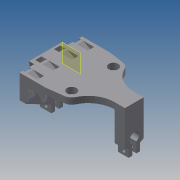
# Autodesk Inventor part: rollerBetter
Saved by Autodesk Inventor 2014 (Build 180170000, 170)
## iProperties
Created: 2014-01-09
Part Number: rollerBetter
Material: Generic
Document SubType Name: Modeling
Designer: Peele
Density: 1 g/cm^3
Appearance: Default
Author: Peele
Autodesk Inventor part; units mm, degrees
ref_plane "YZ Plane" through (0, 0, 0) normal (1, 0, 0) x (0, 1, 0)
ref_plane "XZ Plane" through (0, 0, 0) normal (0, 1, 0) x (-1, 0, 0)
ref_plane "XY Plane" through (0, 0, 0) normal (0, 0, 1) x (1, 0, 0)
sketch "Sketch1" plane through (0, 0, 0) normal (0, 1, 0) x (-1, 0, 0)
  circle A0 centre (0, 20) radius 14.875 construction
  circle A1 centre (0, 20) radius 13.26 construction
  circle A2 centre (0, -20) radius 14.875 construction
  circle A3 centre (0, -20) radius 13.26 construction
  circle A4 centre (0, -20) radius 4.5
  circle A5 centre (0, 20) radius 4.5
  line L0 (0, -20) -> (0, 0) construction
  line L1 (0, 0) -> (0, 20) construction
  arc A6 (-1.036149, 27.932616) -> (-7.232355, 23.419508) centre (0, 20) ccw
  arc A7 (-7.232355, -23.419508) -> (-1.155827, -27.916064) centre (0, -20) ccw
  line L2 (25, 30) -> (40, 30)
  line L3 (40, 30) -> (40, -30)
  line L4 (40, -30) -> (25, -30)
  line L5 (25, -30) -> (25, 30) construction
  line L6 (0, 0) -> (40, 0) construction
  arc A8 (-7.232355, -23.419508) -> (-30, -9) centre (-30, -34.184211) ccw
  arc A9 (-30, 9) -> (-7.232355, 23.419508) centre (-30, 34.184211) ccw
  line L7 (-30, 9) -> (-40, 9)
  line L8 (-40, 9) -> (-40, -9)
  line L9 (-40, -9) -> (-30, -9)
  line L10 (0, 0) -> (-40, 0) construction
  line L11 (25, 30) -> (15, 30)
  arc A10 (15, 30) -> (14.584682, 29.972991) centre (15, 26.793371) ccw
  line L12 (14.584682, 29.972991) -> (-1.036149, 27.932616)
  line L13 (-1.155827, -27.916064) -> (11.253156, -29.727904)
  line L14 (25, -30) -> (15, -30)
  arc A11 (11.253156, -29.727904) -> (15, -30) centre (15, -4.066406) ccw
  dimension "d0" = 29.75
  dimension "d1" = 26.52
  dimension "d2" = 40
  dimension "d3" = 9
  dimension "d4" = 16
  dimension "d5" = 60
  dimension "d6" = 15
  dimension "d7" = 25
  dimension "d66" = 10
  dimension "d67" = 18
  dimension "d68" = 40
  dimension "d87" = 10
  constraints: 30 end point, 13 point on circle, 11 centre point, 11 tangent, 6 coincident, 6 parallel, 3 equal length, 3 equal radius, 3 horizontal, 2 midpoint, 2 perpendicular, 1 collinear, 1 vertical, 4 other
  measures "d0" diameter of A0
  measures "d1" diameter of A1
  measures "d2" distance of point (0, -20) A0.centre
  measures "d3" diameter of A5
  measures "d4" diameter of A6
  measures "d5" distance of L2.end L3.end
  measures "d6" distance of L2.start L2.end
  measures "d7" distance from line of A0.centre L5
  measures "d66" distance of L7.start L7.end
  measures "d67" distance of L7.end L8.end
  measures "d68" distance between parallel lines of L8 L0
  measures "d87" distance of L2.start L11.end
extrude "Extrusion1" add sketch "Sketch1" along normal blind 6
sketch "Sketch2" plane through (0, 0, 0) normal (0, 0, 1) x (1, 0, 0)
  line L0 (-40, 0) -> (-34, 0)
  line L1 (-34, -8.5) -> (-34, -40)
  line L2 (-34, -40) -> (-40, -40)
  line L3 (-40, -40) -> (-40, 0)
  circle A0 centre (-26, -8.5) radius 8
  line L4 (-34, 0) -> (-15.298824, 0)
  line L5 (-15.298824, 0) -> (-18.298824, -10.666076)
  line L6 (7.232355, 0) -> (1.036149, 0)
  point P0 (0, 0)
  point P1 (4.134252, 0)
  dimension "d11" = 6
  dimension "d12" = 40
  dimension "d13" = 16
  dimension "d15" = 8.5
  dimension "d16" = 3
  constraints: 12 end point, 2 parallel, 2 perpendicular, 2 point on circle, 2 tangent, 1 centre point, 1 coincident, 1 horizontal, 1 midpoint
  measures "d11" distance of L1.end L2.end
  measures "d12" distance of L2.end L0.start
  measures "d13" diameter of A0
  measures "d15" distance from line of A0.centre L4
  measures "d16" horizontal distance of L4.end L5.end
extrude "Extrusion11" add sketch "Sketch2" along normal mid plane 60 contours L0 L4 L5 A0 L1 L2 L3
sketch "Sketch11" plane through (0, 0, 0) normal (0, 0, 1) x (1, 0, 0)
  line L0 (40, 0) -> (30, 0)
  line L1 (30, 0) -> (30, -40)
  line L2 (30, -40) -> (40, -40)
  line L3 (40, -40) -> (40, 0)
  line L4 (40, 0) -> (40, 6) projected
  line L5 (-34, -40) -> (-40, -40) projected
  point P0 (0, 0)
  dimension "d71" = 10
  constraints: 8 end point, 2 collinear, 2 parallel, 1 horizontal, 1 perpendicular
  measures "d71" distance of L1.end L2.end
extrude "Extrusion12" add sketch "Sketch11" along normal mid plane 18
sketch "Sketch3" plane through (-25, 6, -30) normal (0, 0, -1) x (-1, 0, 0)
  arc A0 (9, -14.5) -> (-6.701176, -16.666076) centre (1, -14.5) ccw
  arc A1 (7.402553, -13.378697) -> (-5.128468, -16.666076) centre (1, -14.5) ccw
  arc A2 (9, -14.5) -> (-6.701176, -16.666076) centre (1, -14.5) ccw
  line L0 (7.402553, -13.378697) -> (9, -22.5)
  line L1 (9, -22.5) -> (9, -14.5)
  line L2 (-6.701176, -16.666076) -> (-5.128468, -16.666076)
  point P0 (-25, -6)
  point P1 (-5.914822, -16.666076)
  dimension "d74" = 1.5
  dimension "d75" = 8
  constraints: 6 end point, 4 point on circle, 3 tangent, 2 centre point, 2 concentric, 1 coincident, 1 midpoint, 1 perpendicular, 1 point on line, 1 vertical
  measures "d74" radial gap between concentric circles of A0 A1
  measures "d75" distance of L0.end L1.end
extrude "Extrusion13" add sketch "Sketch3" against normal blind 3
mirror "Mirror1" about plane through (0, 0, 0) normal (0, 0, 1) of "Extrusion13"
sketch "Sketch13" plane through (0, 0, 0) normal (0, 0, 1) x (1, 0, 0)
  line L0 (-34, -16.5) -> (-32.402553, -7.378697)
  line L1 (-19.871532, -10.666076) -> (-18.298824, -10.666076)
  line L2 (-18.298824, -10.666076) -> (-15.298824, 0)
  line L3 (-15.298824, 0) -> (-34, 0)
  line L4 (-34, 0) -> (-34, -16.5)
  arc A0 (-19.871532, -10.666076) -> (-32.402553, -7.378697) centre (-26, -8.5) ccw
  arc A1 (-19.871532, -10.666076) -> (-32.402553, -7.378697) centre (-26, -8.5) ccw
  line L5 (-19.871532, -10.666076) -> (-18.298824, -10.666076)
  line L6 (-15.298824, 0) -> (-18.298824, -10.666076)
  line L7 (-15, 0) -> (-15.298824, 0)
  line L8 (-34, -16.5) -> (-34, -40)
  line L9 (-34, -16.5) -> (-32.402553, -7.378697)
  point P0 (0, 0)
  point P1 (-25, 0)
  point P2 (-40, 0)
  constraints: 10 end point, 5 collinear, 2 concentric, 2 point on circle, 1 centre point, 1 horizontal, 1 parallel
extrude "Extrusion14" add sketch "Sketch13" along normal mid plane 4
sketch "Sketch4" plane through (-40, 6, 30) normal (0, 0, 1) x (1, 0, 0)
  arc A0 (20.468886, -13.854567) -> (22.467566, -13.806595) centre (21.467571, -13.80331) ccw
  line L0 (24.701176, -6) -> (21.701176, -16.666076)
  arc A1 (20.128468, -16.666076) -> (7.597447, -13.378697) centre (14, -14.5) ccw
  line L1 (20.468886, -13.854567) -> (16.501696, -13.854567)
  line L2 (16.501696, -13.854567) -> (16.051575, -20.057074)
  line L3 (16.051575, -20.057074) -> (25.203638, -20.057074)
  line L4 (25.203638, -20.057074) -> (25.203638, -13.806595)
  line L5 (25.203638, -13.806595) -> (22.467566, -13.806595)
  point P0 (40, -6)
  dimension "d78" = 1
  constraints: 10 end point, 2 parallel, 2 point on circle, 2 tangent, 1 centre point, 1 horizontal, 1 perpendicular
  measures "d78" radius of A0
sketch "Sketch4 outline for Extrusion4" plane through (-40, 6, 30) normal (0, 0, 1) x (1, 0, 0)
  arc A0 (20.468886, -13.854567) -> (22.467566, -13.806595) centre (21.467571, -13.80331) ccw
  line L0 (22.467566, -13.806595) -> (25.203638, -13.806595)
  line L1 (25.203638, -13.806595) -> (25.203638, -20.057074)
  line L2 (25.203638, -20.057074) -> (16.051575, -20.057074)
  line L3 (16.051575, -20.057074) -> (16.501696, -13.854567)
  line L4 (16.501696, -13.854567) -> (20.468886, -13.854567)
extrude "Extrusion4" cut sketch "Sketch4 outline for Extrusion4" against normal blind 63.8125
sketch "Sketch5" plane through (-40, 6, -30) normal (-1, 0, 0) x (0, 0, 1)
  circle A0 centre (30, -29) radius 4.5
  arc A1 (31.363961, -41.636039) -> (31.363961, -41.636039) centre (41.970563, -52.242641) ccw
  arc A2 (18.636039, -41.636039) -> (18.636039, -41.636039) centre (8.029437, -52.242641) ccw
  line L0 (60, -46) -> (60, 0)
  line L1 (0, 0) -> (60, 0)
  line L2 (0, -46) -> (0, 0)
  line L3 (60, -23) -> (0, -23) construction
  line L4 (30, 0) -> (30, -29) construction
  arc A3 (26.082937, -36.543648) -> (33.917063, -36.543648) centre (30, -29) ccw
  line L5 (0, -23) -> (26.082937, -36.543648)
  line L6 (33.917063, -36.543648) -> (60, -23)
  line L7 (0, -46) -> (60, -46)
  line L8 (0, -23) -> (0, -46)
  line L9 (60, -46) -> (60, -23)
  line L10 (60, -46) -> (0, -46)
  dimension "d28" = 9
  dimension "d81" = 23
  dimension "d82" = 6
  dimension "d83" = 4
  constraints: 14 end point, 6 point on circle, 4 centre point, 4 midpoint, 3 collinear, 2 coincident, 2 tangent, 1 equal length, 1 equal radius, 1 horizontal, 1 vertical
  measures "d28" diameter of A0
  measures "d81" distance between parallel lines of L1 L3
  measures "d82" distance from line of A0.centre L3
  measures "d83" radial gap between concentric circles of A0 A3
extrude "Extrusion15" cut sketch "Sketch5" against normal blind 102.075 contours A0 | L7 A1 | A1 L7 A2 L2 L5 A3 L6 L0 | L7 L2 A2 picked at (45.928029, -45.024991) picked at (13.809124, -44.964168)
sketch "Sketch14" plane through (0, 0, 0) normal (0, 0, 1) x (1, 0, 0)
  line L0 (22, 0) -> (30, 0)
  line L1 (30, 0) -> (30, -14)
  line L2 (30, -14) -> (22, 0)
  line L3 (30, -27.904316) -> (30, 0)
  line L4 (1.155827, 0) -> (-11.253156, 0)
  point P0 (0, 0)
  dimension "d88" = 8
  dimension "d89" = 14
  constraints: 6 end point, 2 collinear, 1 horizontal, 1 perpendicular
  measures "d88" distance of L0.start L0.end
  measures "d89" distance of L0.end L1.end
extrude "Extrusion16" add sketch "Sketch14" along normal mid plane 3
sketch "Sketch6" plane through (-40, 6, -30) normal (-1, 0, 0) x (0, 0, 1)
  line L0 (0, 0) -> (60, 0)
  line L1 (14, 0) -> (46, 0)
  line L2 (46, 0) -> (40, -33.385063)
  line L3 (14, 0) -> (20, -33.385063)
  line L4 (0, -23) -> (26.082937, -36.543648)
  arc A0 (26.082937, -36.543648) -> (33.917063, -36.543648) centre (30, -29) ccw
  line L5 (33.917063, -36.543648) -> (60, -23)
  circle A1 centre (30, -29) radius 4.5
  circle A2 centre (30, -29) radius 4.5
  arc A3 (26.082937, -36.543648) -> (33.917063, -36.543648) centre (30, -29) ccw
  line L6 (33.917063, -36.543648) -> (40, -33.385063)
  line L7 (26.082937, -36.543648) -> (20, -33.385063)
  line L8 (30, -29) -> (30, 0) construction
  point P0 (30, -6)
  dimension "d35" = 32
  dimension "d92" = 20
  constraints: 12 end point, 4 point on line, 4 tangent, 3 point on circle, 2 centre point, 2 concentric, 1 coincident, 1 collinear, 1 equal length, 1 midpoint, 1 vertical
  measures "d35" distance of L1.start L1.end
  measures "d92" distance of L2.end L3.end
extrude "Extrusion17" add sketch "Sketch6" along normal blind 5
sketch "Sketch15" plane through (-45, 6, -30) normal (-1, 0, 0) x (0, 0, 1)
  arc A0 (26.082937, -36.543648) -> (33.917063, -36.543648) centre (30, -29) ccw
  line L0 (28, -58.774006) -> (32, -58.774006)
  line L1 (32, -58.774006) -> (32, -29)
  line L2 (32, -29) -> (28, -29)
  line L3 (28, -29) -> (28, -58.774006)
  line L4 (28, -58.774006) -> (32, -29) construction
  line L5 (32, -58.774006) -> (28, -29) construction
  line L6 (30, -29) -> (30, -43.887003) construction
  point P0 (30, -6)
  dimension "d95" = 4
  constraints: 14 end point, 3 midpoint, 3 parallel, 1 coincident, 1 horizontal, 1 perpendicular
  measures "d95" distance of L0.start L0.end
extrude "Extrusion18" cut sketch "Sketch15" against normal blind 103.425
sketch "Sketch16" plane through (-45, 6, -30) normal (-1, 0, 0) x (0, 0, 1)
  line L0 (28, -33.031129) -> (24.5, -33.031129)
  line L1 (24.5, -33.031129) -> (24.5, -43.031129)
  line L2 (24.5, -43.031129) -> (28, -43.031129)
  line L3 (28, -43.031129) -> (28, -33.031129)
  line L4 (32, -33.031129) -> (35.5, -33.031129)
  line L5 (35.5, -33.031129) -> (35.5, -43.031129)
  line L6 (35.5, -43.031129) -> (32, -43.031129)
  line L7 (32, -43.031129) -> (32, -33.031129)
  point P0 (30, -6)
  dimension "d98" = 3.5
  dimension "d99" = 10
  constraints: 16 end point, 4 parallel, 2 collinear, 2 horizontal, 2 perpendicular
  measures "d98" distance of L1.end L2.end
  measures "d99" distance of L0.end L1.end
extrude "Extrusion19" add sketch "Sketch16" against normal up to surface (11 mm away)
sketch "Sketch17" plane through (40, 6, 9) normal (1, 0, 0) x (0, 0, -1)
  line L0 (7, -33.031129) -> (3.5, -33.031129)
  line L1 (3.5, -33.031129) -> (3.5, -43.031129)
  line L2 (3.5, -43.031129) -> (7, -43.031129)
  line L3 (7, -43.031129) -> (7, -33.031129)
  line L4 (11, -33.031129) -> (14.5, -33.031129)
  line L5 (14.5, -33.031129) -> (14.5, -43.031129)
  line L6 (14.5, -43.031129) -> (11, -43.031129)
  line L7 (11, -43.031129) -> (11, -33.031129)
  point P0 (9, -6)
  constraints: 16 end point, 4 parallel, 2 equal length, 2 horizontal, 2 perpendicular, 1 coincident
extrude "Extrusion20" add sketch "Sketch17" against normal up to surface (10 mm away)
sketch "Sketch18" plane through (-45, -37.031129, -5.5) normal (0, 0, -1) x (-1, 0, 0)
  line L0 (-11, 7.309426) -> (-11, 0)
  line L1 (0, 0) -> (-11, 0)
  line L2 (0, 7.309426) -> (0, 0)
  circle A0 centre (-5.5, 3.654713) radius 1.675
  circle A1 centre (-80, 3.654713) radius 1.675
  line L3 (-5.5, 0) -> (-5.5, 3.654713) construction
  line L4 (-80, 3.654713) -> (-80, 0) construction
  line L5 (0, 3.654713) -> (-5.5, 3.654713) construction
  line L6 (-80, 3.654713) -> (-5.5, 3.654713) construction
  line L7 (-85, 7.309426) -> (-85, 9.126812)
  point P0 (-45, 37.031129)
  dimension "d106" = 3.35
  dimension "d107" = 5
  constraints: 8 end point, 2 centre point, 2 midpoint, 2 parallel, 1 collinear, 1 equal radius, 1 perpendicular, 1 vertical
  measures "d106" diameter of A1
  measures "d107" distance between parallel lines of L4 L7
extrude "Extrusion21" cut sketch "Sketch18" against normal blind 103.425
sketch "Sketch19" plane through (-34, -16.5, 27) normal (0, 0, -1) x (-1, 0, 0)
  arc A0 (0, 8) -> (-15.998581, 7.849324) centre (-8, 8) ccw
  arc A1 (5.617699, 18.034513) -> (1.59339, 22.149801) centre (3, 19.5) ccw
  line L0 (1.59339, 22.149801) -> (-11.750961, 15.066137)
  line L1 (6, 22.5) -> (-19, 22.5)
  line L2 (6, -0.5) -> (6, 22.5)
  line L3 (5.617699, 18.034513) -> (0, 8)
  line L4 (-23.608822, 14.432357) -> (8.880546, 31.67889)
  line L5 (8.880546, 31.67889) -> (14.828162, 31.67889)
  line L6 (14.828162, 31.67889) -> (13.156758, 25.359716)
  line L7 (13.156758, 25.359716) -> (-1.745133, -1.258516)
  line L8 (-1.745133, -1.258516) -> (0, 8)
  line L9 (-11.750961, 15.066137) -> (-11.750961, 3.402667)
  line L10 (-11.750961, 3.402667) -> (-23.608822, 6.539038)
  line L11 (-23.608822, 6.539038) -> (-23.608822, 14.432357)
  point P0 (-34, 16.5)
  dimension "d111" = 3
  dimension "d112" = 5
  dimension "d113" = 3
  constraints: 20 end point, 5 tangent, 3 parallel, 3 perpendicular, 3 point on circle, 1 centre point
  measures "d111" radius of A1
  measures "d112" distance between parallel lines of L4 L0
  measures "d113" distance between parallel lines of L7 L3
extrude "Extrusion22" cut sketch "Sketch19" along normal blind 6 contours L3 A1 L2 L7 L8 | L9 L10 L11 L4 L1 A1 L0 | L2 L1 L4 L5 L6 L7 | A1 L1 L2
ref_plane "Work Plane1" through (0, 0, 6) normal (0, 0, 1) x (1, 0, 0)
sketch "Sketch21" plane through (0, 0, 6) normal (0, 0, 1) x (1, 0, 0)
  line L0 (-40, 6) -> (-45, 6) construction
  line L1 (-45, 6) -> (-45, -27.385063) construction
  line L2 (-35.59339, 5.649801) -> (-22.249039, -1.433863)
  line L3 (-34, -14.641304) -> (-43, 1.434783)
  line L4 (-43, 1.434783) -> (-43, 15.2423)
  line L5 (-43, 15.2423) -> (-14.286246, 0)
  line L6 (-14.286246, 0) -> (-14.286246, -19.159136)
  arc A0 (-18.001419, -8.650676) -> (-34, -8.5) centre (-26, -8.5) ccw construction
  line L7 (1.155827, 0) -> (-11.253156, 0) construction
  line L8 (-22.249039, -1.433863) -> (-22.249039, -19.159136)
  line L9 (-22.249039, -19.159136) -> (-14.286246, -19.159136)
  line L10 (-39.617699, 1.534513) -> (-34, -8.5)
  line L11 (-34, -8.5) -> (-34, -14.641304)
  arc A1 (-35.59339, 5.649801) -> (-39.617699, 1.534513) centre (-37, 3) ccw
  line L12 (-40, -27.385063) -> (-40, 6)
  point P0 (0, 0)
  dimension "d119" = 5
  dimension "d123" = 3
  dimension "d126" = 3
  dimension "d127" = 2
  constraints: 18 end point, 6 tangent, 4 parallel, 3 perpendicular, 3 point on circle, 1 centre point, 1 point on line
  measures "d119" distance between parallel lines of L5 L2
  measures "d123" distance between parallel lines of L3 L10
  measures "d126" radius of A1
  measures "d127" distance between parallel lines of L1 L4
extrude "Extrusion24" cut sketch "Sketch21" along normal blind 6
mirror "Mirror2" about plane through (0, 0, 0) normal (0, 0, 1) of "Extrusion24", "Extrusion22"
body "Solid1"
